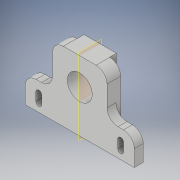
# Autodesk Inventor part: OldhamCouplerTop
Saved by Autodesk Inventor 2018 (Build 220112000, 112)
## iProperties
Created: 2017-10-05
Part Number: OldhamCouplerTop
Material: Generic
Document SubType Name: Modeling
Designer: Jurjen
Density: 1 g/cm^3
Appearance: Default
Author: Jurjen
Autodesk Inventor part; units mm, degrees
ref_plane "XZ Plane" through (0, 0, 0) normal (0, 1, 0) x (-1, 0, 0)
ref_plane "XY Plane" through (0, 0, 0) normal (0, 0, 1) x (1, 0, 0)
sketch "Sketch1" plane through (0, 0, 0) normal (0, 0, 1) x (1, 0, 0)
  line L0 (-20, 31) -> (20, 31)
  line L1 (20, 31) -> (20, 0)
  line L2 (-20, 0) -> (-20, 31)
  line L3 (40, 0) -> (40, -20)
  line L4 (40, -20) -> (-40, -20)
  line L5 (-40, -20) -> (-40, 0)
  line L6 (-40, 0) -> (-20, 0)
  line L7 (20, 0) -> (40, 0)
  circle A0 centre (0, 11) radius 9.125
  point P0 (0, 0)
  point P1 (0, 31)
  point P2 (0, -20)
  dimension "d0" = 80
  dimension "d1" = 20
  dimension "d2" = 40
  dimension "d3" = 31
  dimension "d6" = 18.25
  dimension "d7" = 20
  constraints: 16 end point, 4 parallel, 3 horizontal, 3 perpendicular, 3 vertical alignment, 2 horizontal alignment, 2 midpoint, 1 centre point
  measures "d0" distance of L3.end L4.end
  measures "d1" distance of L3.start L3.end
  measures "d2" distance of L0.start L0.end
  measures "d3" distance of L0.end L1.end
  measures "d6" diameter of A0
  measures "d7" distance from line of L0 A0.centre
extrude "Extrusion1" add sketch "Sketch1" along normal blind 6.5 contours L0 L1 L7 L3 L4 L5 L6 L2 | A0
sketch "Sketch2" plane through (0, 0, 6.5) normal (0, 0, 1) x (1, 0, 0)
  circle A0 centre (0, 11) radius 9.125
  line L0 (20, 31) -> (-20, 31) projected
  point P0 (0, 0)
  dimension "d8" = 20
  dimension "d9" = 18.25
  constraints: 1 centre point
  measures "d8" distance from line of L0 A0.centre
  measures "d9" diameter of A0
sketch "Sketch3" plane through (0, 0, 0) normal (0, 0, -1) x (-1, 0, 0)
  line L0 (-20, 31) -> (20, 31) projected
  line L1 (40, -20) -> (-40, -20) projected
  line L2 (20, 31) -> (-20, 31)
  line L3 (-20, 31) -> (-20, -20)
  line L4 (-20, -20) -> (20, -20)
  line L5 (20, -20) -> (20, 31)
  point P0 (0, 0)
  point P1 (-20, 5.5)
  point P2 (-20, 0)
  constraints: 8 end point, 2 parallel, 1 horizontal, 1 midpoint, 1 perpendicular, 1 point on line, 1 vertical alignment
extrude "Extrusion2" add sketch "Sketch3" along normal blind 3.5
sketch "Sketch4" plane through (0, 0, -3.5) normal (0, 0, -1) x (-1, 0, 0)
  line L0 (-20, 31) -> (20, 31) projected
  line L1 (-20, -20) -> (20, -20) projected
  line L2 (11.85, 31) -> (-11.85, 31)
  line L3 (-11.85, 31) -> (-11.85, -20)
  line L4 (-11.85, -20) -> (11.85, -20)
  line L5 (11.85, -20) -> (11.85, 31)
  point P0 (0, 0)
  point P1 (0, 31)
  dimension "d12" = 23.7
  constraints: 8 end point, 2 parallel, 2 point on line, 1 horizontal, 1 midpoint, 1 perpendicular, 1 vertical alignment
  measures "d12" distance between parallel lines of L3 L5
extrude "Extrusion3" add sketch "Sketch4" along normal blind 5
extrude "Extrusion4" cut sketch "Sketch2" against normal up to next
fillet "Fillet1" radius 8 6 edges at (-20, 31, 1.5) (-40, 0, 3.25) (20, 31, 1.5) (-20, 0, 3.25) (40, 0, 3.25) (20, 0, 3.25)
sketch "Sketch5" plane through (0, 0, 0) normal (0, 0, -1) x (-1, 0, 0)
  arc A0 (27.9, -14) -> (32.1, -14) centre (30, -14) ccw
  arc A1 (32.1, -7.88) -> (27.9, -7.88) centre (30, -7.88) ccw
  line L0 (32.1, -7.88) -> (32.1, -14)
  line L1 (27.9, -7.88) -> (27.9, -14)
  line L2 (40, -20) -> (40, -8) projected
  line L3 (20, -20) -> (40, -20) projected
  point P0 (0, 0)
  dimension "d18" = 4.2
  dimension "d19" = 6.12
  dimension "d20" = 10
  dimension "d21" = 6
  constraints: 4 end point, 4 point on circle, 3 tangent, 2 centre point, 2 vertical, 1 equal radius
  measures "d18" diameter of A1
  measures "d19" distance of L0.start L0.end
  measures "d20" distance from line of L2 A0.centre
  measures "d21" distance from line of L3 A0.centre
extrude "Extrusion5" cut sketch "Sketch5" against normal up to next
mirror "Mirror1" about plane through (0, 0, 0) normal (1, 0, 0) of "Extrusion5"
body "Solid1"
